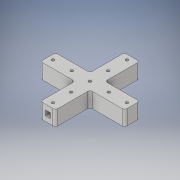
# Autodesk Inventor part: main
Saved by Autodesk Inventor 2019 (Build 230136000, 136)
## iProperties
Created: 2019-03-09
Part Number: main
Material: Generic
Document SubType Name: Modeling
Designer: Jaden
Density: 1 g/cm^3
Appearance: Default
Author: Jaden
Autodesk Inventor part; units mm, degrees
ref_plane "YZ Plane" through (0, 0, 0) normal (1, 0, 0) x (0, 1, 0)
ref_plane "XZ Plane" through (0, 0, 0) normal (0, 1, 0) x (-1, 0, 0)
ref_plane "XY Plane" through (0, 0, 0) normal (0, 0, 1) x (1, 0, 0)
sketch "Sketch1" plane through (0, 0, 0) normal (0, 1, 0) x (-1, 0, 0)
  line L0 (6.35, 53.34) -> (-6.35, 53.34)
  arc A0 (9.525, 50.165) -> (6.35, 53.34) centre (6.35, 50.165) ccw
  arc A1 (-6.35, 53.34) -> (-9.525, 50.165) centre (-6.35, 50.165) ccw
  line L1 (6.35, -53.34) -> (-6.35, -53.34)
  arc A2 (6.35, -53.34) -> (9.525, -50.165) centre (6.35, -50.165) ccw
  arc A3 (-9.525, -50.165) -> (-6.35, -53.34) centre (-6.35, -50.165) ccw
  line L2 (-53.34, 6.35) -> (-53.34, -6.35)
  line L3 (53.34, 6.35) -> (53.34, -6.35)
  arc A4 (53.34, 6.35) -> (50.165, 9.525) centre (50.165, 6.35) ccw
  arc A5 (50.165, -9.525) -> (53.34, -6.35) centre (50.165, -6.35) ccw
  arc A6 (-50.165, 9.525) -> (-53.34, 6.35) centre (-50.165, 6.35) ccw
  arc A7 (-53.34, -6.35) -> (-50.165, -9.525) centre (-50.165, -6.35) ccw
  line L4 (9.525, 50.165) -> (9.525, 12.7)
  line L5 (9.525, -12.7) -> (9.525, -50.165)
  line L6 (50.165, 9.525) -> (12.7, 9.525)
  line L7 (-12.7, 9.525) -> (-50.165, 9.525)
  line L8 (-9.525, -50.165) -> (-9.525, -12.7)
  line L9 (-9.525, 12.7) -> (-9.525, 50.165)
  line L10 (50.165, -9.525) -> (12.7, -9.525)
  line L11 (-12.7, -9.525) -> (-50.165, -9.525)
  circle A8 centre (46.99, 0) radius 1.7
  circle A9 centre (-46.99, 0) radius 1.7
  circle A10 centre (0, 46.99) radius 1.7
  circle A11 centre (0, -46.99) radius 1.7
  circle A12 centre (0, 0) radius 1.7
  circle A13 centre (0, 23.9395) radius 1.7
  circle A14 centre (0, -23.0505) radius 1.7
  circle A15 centre (23.0505, 0) radius 1.7
  circle A16 centre (-23.9395, 0) radius 1.7
  arc A17 (9.525, 12.7) -> (12.7, 9.525) centre (12.7, 12.7) ccw
  arc A18 (-12.7, 9.525) -> (-9.525, 12.7) centre (-12.7, 12.7) ccw
  arc A19 (12.7, -9.525) -> (9.525, -12.7) centre (12.7, -12.7) ccw
  arc A20 (-9.525, -12.7) -> (-12.7, -9.525) centre (-12.7, -12.7) ccw
  point P0 (9.525, 53.34)
  point P1 (9.525, -53.34)
  point P2 (-9.525, -53.34)
  point P3 (-9.525, 53.34)
  point P4 (53.34, 9.525)
  point P5 (-53.34, 9.525)
  point P6 (53.34, -9.525)
  point P7 (-53.34, -9.525)
  dimension "d0" = 106.68
  dimension "d1" = 53.34
  dimension "d3" = 106.68
  dimension "d5" = 3.175
  dimension "d6" = 3.175
  dimension "d7" = 106.68
  dimension "d8" = 53.34
  dimension "d10" = 106.68
  dimension "d11" = 53.34
  dimension "d13" = 3.175
  dimension "d14" = 3.4
  dimension "d15" = 3.4
  dimension "d16" = 93.98
  dimension "d17" = 46.99
  dimension "d18" = 3.4
  dimension "d19" = 3.4
  dimension "d20" = 93.98
  dimension "d21" = 46.99
  dimension "d22" = 3.4
  dimension "d23" = 3.4
  dimension "d24" = 23.9395
  dimension "d25" = 3.4
  dimension "d26" = 46.99
  dimension "d27" = 3.4
  dimension "d28" = 3.4
  dimension "d29" = 23.9395
  dimension "d30" = 46.99
  dimension "d31" = 3.175
  constraints: 32 tangent, 24 end point, 24 point on circle, 21 centre point, 8 equal radius, 8 point on line, 5 horizontal, 4 vertical, 1 coincident
  measures "d0" distance of point (9.525, 53.34) point (9.525, -53.34)
  measures "d1" vertical distance of point (0, 0) point (9.525, -53.34)
  measures "d3" distance of point (-9.525, -53.34) point (-9.525, 53.34)
  measures "d5" radius of A0
  measures "d6" radius of A2
  measures "d7" distance of point (53.34, 9.525) point (-53.34, 9.525)
  measures "d8" horizontal distance of point (0, 0) point (53.34, 9.525)
  measures "d10" distance of point (53.34, -9.525) point (-53.34, -9.525)
  measures "d11" horizontal distance of point (0, 0) point (53.34, -9.525)
  measures "d13" radius of A4
  measures "d14" diameter of A8
  measures "d15" diameter of A9
  measures "d16" distance of A8.centre A9.centre
  measures "d17" distance of point (0, 0) A9.centre
  measures "d18" diameter of A10
  measures "d19" diameter of A11
  measures "d20" distance of A11.centre A10.centre
  measures "d21" distance of point (0, 0) A11.centre
  measures "d22" diameter of A12
  measures "d23" diameter of A13
  measures "d24" distance of point (0, 0) A13.centre
  measures "d25" diameter of A14
  measures "d26" distance of A14.centre A13.centre
  measures "d27" diameter of A15
  measures "d28" diameter of A16
  measures "d29" distance of point (0, 0) A16.centre
  measures "d30" distance of A15.centre A16.centre
  measures "d31" radius of A17
extrude "Extrusion1" add sketch "Sketch1" along normal blind 19.05
sketch "Sketch2" plane through (-6.35, 0, 53.34) normal (0, 0, 1) x (1, 0, 0)
  line L0 (3.1242, 6.2992) -> (9.5758, 6.2992)
  line L1 (9.5758, 6.2992) -> (9.5758, 12.7508)
  line L2 (9.5758, 12.7508) -> (3.1242, 12.7508)
  line L3 (3.1242, 12.7508) -> (3.1242, 6.2992)
  line L4 (3.1242, 6.2992) -> (9.5758, 12.7508) construction
  line L5 (9.5758, 6.2992) -> (3.1242, 12.7508) construction
  line L6 (0, 19.05) -> (12.7, 19.05) projected
  line L7 (15.875, 0) -> (15.875, 19.05) projected
  point P0 (6.35, 0)
  point P1 (6.35, 9.525)
  dimension "d34" = 6.4516
  dimension "d35" = 6.4516
  dimension "d36" = 9.525
  dimension "d37" = 9.525
  constraints: 12 end point, 2 midpoint, 2 parallel, 1 horizontal, 1 perpendicular
  measures "d34" distance of L2.end L1.end
  measures "d35" distance of L1.end L0.end
  measures "d36" distance from line of L6 point (6.35, 9.525)
  measures "d37" distance from line of L7 point (6.35, 9.525)
extrude "Extrusion2" cut sketch "Sketch2" against normal through all
body "Solid1"
